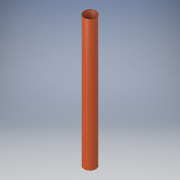
# Autodesk Inventor part: 8 in Phenolic Linter
Saved by Autodesk Inventor 2017 (Build 210142000, 142)
## iProperties
Created: 2016-07-18
Part Number: 8 in Phenolic Linter
Material: Phenolic Resin
Document SubType Name: Modeling
Designer: Monique
Density: 1.38 g/cm^3
Appearance: Smooth - Light Orange
Author: Monique
Autodesk Inventor part; units mm, degrees
ref_plane "YZ Plane" through (0, 0, 0) normal (1, 0, 0) x (0, 1, 0)
ref_plane "XZ Plane" through (0, 0, 0) normal (0, 1, 0) x (-1, 0, 0)
ref_plane "XY Plane" through (0, 0, 0) normal (0, 0, 1) x (1, 0, 0)
sketch "Sketch1" plane through (0, 0, 0) normal (0, 1, 0) x (-1, 0, 0)
  circle A0 centre (0, 0) radius 95.25
  circle A1 centre (0, -1.2289) radius 92.075
  dimension "d0" = 190.5
  dimension "d1" = 184.15
  constraints: 2 centre point, 1 coincident
  measures "d0" diameter of A0
  measures "d1" diameter of A1
extrude "Extrusion1" add sketch "Sketch1" along normal blind 2133.6
body "Solid1"
